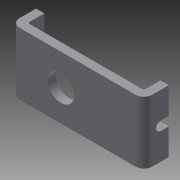
# Autodesk Inventor part: Base-Plate
Saved by Autodesk Inventor 2015 SP2 (Build 190223200, 223)
## iProperties
Created: 2015-12-04
Part Number: Base-Plate
Material: Generic
Document SubType Name: Sheet Metal
Designer: KC-019
Density: 1 g/cm^3
Sheet Metal Rule: Default_mm
Appearance: Default
Author: KC-019
Autodesk Inventor part; units mm, degrees
ref_plane "YZ Plane" through (0, 0, 0) normal (1, 0, 0) x (0, 1, 0)
ref_plane "XZ Plane" through (0, 0, 0) normal (0, 1, 0) x (-1, 0, 0)
ref_plane "XY Plane" through (0, 0, 0) normal (0, 0, 1) x (1, 0, 0)
sketch "Sketch1" plane through (0, 0, 0) normal (0, 0, 1) x (1, 0, 0)
  line L0 (10, 0) -> (150, 0)
  line L1 (160, 0) -> (160, 30)
  line L2 (0, 10) -> (0, 30)
  line L3 (0, 30) -> (10, 30)
  line L4 (10, 30) -> (10, 10)
  line L5 (12, 10) -> (150, 10)
  line L6 (150, 12) -> (150, 30)
  line L7 (150, 30) -> (160, 30)
  arc A0 (0, 10) -> (10, 0) centre (10, 10) ccw
  arc A1 (150, 0) -> (160, 10) centre (150, 10) ccw
  arc A2 (10, 12) -> (12, 10) centre (12, 12) ccw
  arc A3 (148, 10) -> (150, 12) centre (148, 12) ccw
  point P0 (0, 0)
  dimension "d0" = 160
  dimension "d1" = 30
  dimension "d2" = 30
  dimension "d3" = 10
  dimension "d4" = 20
  dimension "d5" = 140
  dimension "d8" = 20
  dimension "d9" = 20
  dimension "d10" = 4
  dimension "d11" = 4
  constraints: 16 end point, 8 point on circle, 8 tangent, 5 perpendicular, 4 centre point, 4 point on line, 4 vertical, 3 horizontal
  measures "d0" distance of point (0, 0) L1.start
  measures "d1" distance of L1.start L1.end
  measures "d2" distance of point (0, 0) L2.end
  measures "d3" distance of L2.end L3.end
  measures "d4" distance of L3.end L4.end
  measures "d5" distance of L4.end L5.end
  measures "d8" diameter of A0
  measures "d9" diameter of A1
  measures "d10" diameter of A2
  measures "d11" diameter of A3
extrude "Extrusion1" add sketch "Sketch1" along normal mid plane 75
sketch "Sketch2" plane through (160, 10, 37.5) normal (1, 0, 0) x (0, 0, -1)
  line L0 (37.5, -10) -> (0, -10)
  line L1 (0, -10) -> (75, -10) projected
  line L2 (32, 20) -> (32, 10)
  line L3 (43, 20) -> (43, 10)
  arc A0 (32, 10) -> (43, 10) centre (37.5, 10) ccw
  line L4 (32, 20) -> (43, 20)
  line L5 (75, 20) -> (0, 20) projected
  dimension "d16" = 11
  constraints: 8 end point, 2 collinear, 2 point on circle, 2 vertical, 1 centre point, 1 other
  measures "d16" distance of L3.start L2.start
extrude "Extrusion2" cut sketch "Sketch2" against normal blind 75
sketch "Sketch3" plane through (12, 10, 37.5) normal (0, 1, 0) x (1, 0, 0)
  line L0 (0, 0) -> (0, 75) projected
  circle A0 centre (48, 37.5) radius 16
  line L1 (-12, 0) -> (-12, 75) projected
  line L2 (-12, 0) -> (-12, 37.5)
  line L3 (-12, 37.5) -> (48, 37.5)
  dimension "d20" = 32
  dimension "d22" = 60
  constraints: 4 end point, 1 centre point, 1 coincident, 1 collinear, 1 perpendicular
  measures "d20" diameter of A0
  measures "d22" distance of L2.end L3.end
extrude "Extrusion3" cut sketch "Sketch3" against normal through all
equation "\"BendRadius\" = Thickness"
equation "\"BendReliefWidth\" = Thickness"
equation "\"BendReliefDepth\" = 0.5 * Thickness"
equation "\"CornerReliefSize\" = 4 * Thickness"
equation "\"MinimumRemnant\" = 2 * Thickness"
equation "\"TransitionRadius\" = BendRadius"
equation "\"JacobiRadiusSize\" = BendRadius"
equation "\"GapSize\" = Thickness"
equation "\"Thickness\" = 0.5"
body "Solid1"
